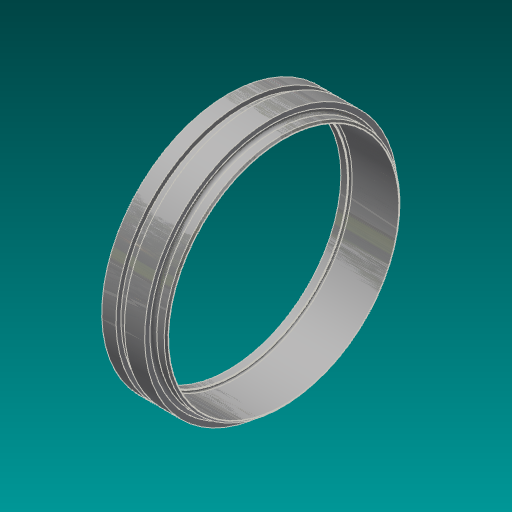
# Autodesk Inventor part: A1-19027-400-05 34in Type B Victaulic ring
Saved by Autodesk Inventor 2017.3 (Build 213257000, 257)
## iProperties
Created: 2014-07-03
Part Number: A1-19027-400-05 34in Type B Victaulic ring
Material: Steel, Mild
Document SubType Name: Modeling
Designer: Graeme_Van_Dongen
Density: 7.86 g/cm^3
Appearance: Steel
Description: 34" TYPE B VICTAULIC RING FOR STYLE 2xx COUPLING - CUSTOM, A105N
Mass: 148308 g
Surface Area: 14322.5 cm^2
Volume: 18868.7 cm^3
Author: Graeme_Van_Dongen
Autodesk Inventor part; units mm, degrees
ref_plane "YZ Plane" through (0, 0, 0) normal (1, 0, 0) x (0, 1, 0)
ref_plane "XZ Plane" through (0, 0, 0) normal (0, 1, 0) x (-1, 0, 0)
ref_plane "XY Plane" through (0, 0, 0) normal (0, 0, 1) x (1, 0, 0)
sketch "Sketch1" plane through (0, 0, 0) normal (0, 0, 1) x (1, 0, 0)
  line L0 (0, 412.75) -> (0, 463.55)
  line L1 (0, 463.55) -> (52.07, 463.55)
  line L2 (52.07, 463.55) -> (54.7572, 448.31)
  line L3 (54.7572, 448.31) -> (77.4902, 448.31)
  line L4 (77.4902, 448.31) -> (83.0371, 463.55)
  line L5 (83.0371, 463.55) -> (157.1625, 463.55)
  line L6 (169.8625, 431.8) -> (197.1093, 431.8)
  line L7 (197.1093, 431.8) -> (203.2, 423.8625)
  line L8 (203.2, 422.275) -> (157.1625, 422.275)
  line L9 (25.4, 415.925) -> (25.4, 412.75)
  line L10 (25.4, 412.75) -> (0, 412.75)
  arc A0 (31.75, 422.275) -> (25.4, 415.925) centre (31.75, 415.925) ccw
  line L11 (-40.64, 0) -> (243.84, 0) projected
  line L12 (203.2, 422.275) -> (203.2, 423.8625)
  line L13 (31.75, 422.275) -> (157.1625, 422.275)
  line L14 (157.1625, 463.55) -> (157.1625, 444.5)
  arc A1 (157.1625, 444.5) -> (169.8625, 431.8) centre (169.8625, 444.5) ccw
  point P0 (0, 0)
  dimension "d0" = 463.55
  dimension "d3" = 431.8
  dimension "d5" = 7.9375
  dimension "d10" = 6.35
  dimension "d12" = 412.75
  dimension "d13" = 52.07
  dimension "d17" = 9.525
  dimension "d35" = 25.4
  dimension "d38" = 10
  dimension "d39" = 20
  dimension "d40" = 22.733
  dimension "d41" = 15.24
  dimension "d44" = 203.2
  dimension "d45" = 37.5
  dimension "d55" = 422.275
  dimension "d58" = 12.7
  dimension "d59" = 157.1625
  constraints: 29 end point, 5 parallel, 4 point on circle, 4 tangent, 3 vertical, 2 centre point, 2 collinear, 2 point on line, 1 horizontal, 1 perpendicular
  measures "d0" distance from line of point (0, 0) L1
  measures "d3" distance from line of point (0, 0) L6
  measures "d5" vertical distance of L7.end L6.end
  measures "d10" radius of A0
  measures "d12" distance from line of point (0, 0) L10
  measures "d13" distance of L0.end L1.end
  measures "d17" distance between parallel lines of L10 L8
  measures "d35" distance between parallel lines of L9 L0
  measures "d38" angle of L0 L2
  measures "d39" angle of L0 L4
  measures "d40" distance of L2.end L3.end
  measures "d41" distance between parallel lines of L1 L3
  measures "d44" distance between parallel lines of L12 L0
  measures "d45" angle of L12 L7
  measures "d55" distance between parallel lines of L11 L13
  measures "d58" radius of A1
  measures "d59" distance between parallel lines of L14 L0
revolve "Revolution1" add sketch "Sketch1" angle 360 about axis through (-10, 0, 0) along (1, 0, 0)
chamfer "Chamfer2" distance 0.7937 angle 45 1 edges at (25.4, -412.75, 0)
body "Solid1"
